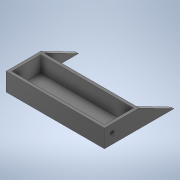
# Autodesk Inventor part: BodyWedgeV1-NoMotor
Saved by Autodesk Inventor 2020 (Build 240168000, 168)
## iProperties
Created: 2023-11-26
Part Number: BodyWedgeV1-NoMotor
Material: Thermoplastic Resin
Document SubType Name: Modeling
Designer: smz3rm
Density: 1.28 g/cm^3
Appearance: Smooth - Black
Mass: 129.558 g
Surface Area: 511.807 cm^2
Volume: 101.217 cm^3
Author: smz3rm
Autodesk Inventor part; units mm, degrees
ref_plane "YZ Plane" through (0, 0, 0) normal (1, 0, 0) x (0, 1, 0)
ref_plane "XZ Plane" through (0, 0, 0) normal (0, 1, 0) x (-1, 0, 0)
ref_plane "XY Plane" through (0, 0, 0) normal (0, 0, 1) x (1, 0, 0)
sketch "Sketch1" plane through (0, 0, 0) normal (0, 1, 0) x (-1, 0, 0)
  line L0 (85, 30) -> (-85, 30)
  line L1 (-85, 30) -> (-85, -30)
  line L2 (-85, -30) -> (85, -30)
  line L3 (85, -30) -> (85, 30)
  line L4 (85, 30) -> (-85, -30) construction
  line L5 (-85, 30) -> (85, -30) construction
  line L6 (0, -42) -> (0, 42) projected
  point P0 (0, 0)
  point P1 (-100, -30)
  point P2 (-85, -27)
  dimension "d0" = 170
  dimension "d1" = 60
  dimension "d32" = 15
  constraints: 12 end point, 2 midpoint, 2 parallel, 2 point on line, 1 horizontal, 1 perpendicular
  measures "d0" distance of L2.end L1.end
  measures "d1" distance of L1.end L0.end
  measures "d32" distance of L1.end point (-100, -30)
extrude "Extrusion1" add sketch "Sketch1" along normal blind 3
sketch "Sketch2" plane through (0, 3, 0) normal (0, 1, 0) x (1, 0, 0)
  line L0 (-85, 30) -> (-85, -30) projected
  line L1 (-85, -30) -> (85, -30) projected
  line L2 (85, -30) -> (85, 30) projected
  line L3 (80, -25) -> (-80, -25)
  line L4 (-80, -25) -> (-80, 25)
  line L5 (-80, 25) -> (80, 25)
  line L6 (80, 25) -> (80, -25)
  line L7 (80, -25) -> (-80, 25) construction
  line L8 (-80, -25) -> (80, 25) construction
  line L9 (85, 30) -> (-85, 30) projected
  point P0 (0, 0)
  dimension "d36" = 160
  dimension "d37" = 50
  constraints: 12 end point, 2 midpoint, 2 parallel, 1 horizontal, 1 perpendicular
  measures "d36" distance of L4.end L5.end
  measures "d37" distance between parallel lines of L5 L3
extrude "Extrusion2" add sketch "Sketch2" along normal blind 28
sketch "Sketch9" plane through (-80, 20, 19) normal (1, 0, 0) x (0, 0, -1)
  circle A0 centre (2, -3) radius 3.5
  line L0 (49, -20) -> (-11, -20) projected
  line L1 (-11, -20) -> (-11, 11) projected
  point P0 (19, -20)
  point P1 (44, -20)
  dimension "d27" = 7
  dimension "d28" = 17
  dimension "d41" = 13
  constraints: 1 centre point
  measures "d27" diameter of A0
  measures "d28" distance from line of L0 A0.centre
  measures "d41" distance from line of L1 A0.centre
extrude "Extrusion7" cut sketch "Sketch9" against normal up to surface (5 mm away)
mirror "Mirror2" about plane through (0, 0, 0) normal (1, 0, 0) of "Extrusion7"
sketch "Sketch14" plane through (0, 3, 0) normal (0, 1, 0) x (1, 0, 0)
  point P0 (0, 0)
sketch "Sketch15" plane through (85, 0, 30) normal (1, 0, 0) x (0, 0, -1)
  line L0 (60, 31) -> (0, 31) projected
  line L1 (60, 31) -> (120, 0)
  line L2 (120, 0) -> (60, 0)
  circle A0 centre (13, 17) radius 3.5 projected
  line L3 (0, 0) -> (60, 0) projected
  line L4 (60, 0) -> (60, 31) projected
  line L5 (0, 31) -> (60, 31) projected
  line L6 (0, 0) -> (0, 31) projected
  point P0 (30, 0)
  dimension "d67" = 60
  constraints: 4 end point, 1 parallel
  measures "d67" distance of L2.end L1.end
extrude "Extrusion12" add sketch "Sketch15" against normal blind 5 contours L1 L2 L4
mirror "Mirror5" about plane through (0, 0, 0) normal (1, 0, 0) of "Extrusion12"
equation "\"d0\" = Width"
equation "\"d1\" = Length"
equation "\"d32\" = -0.5 * Width + 0.5 * FullWidth"
equation "\"d2\" = BaseWallThickness"
equation "\"d36\" = Width - 2 * SideWallThickness"
equation "\"d37\" = Length - 2 * SideWallThickness"
equation "\"d5\" = Height - 2 * BaseWallThickness"
equation "\"d28\" = DriveMotorHeight"
equation "\"d67\" = WedgeLength"
equation "\"d68\" = SideWallThickness"
equation "\"SideWallThickness\" = 5"
equation "\"BaseWallThickness\" = 3"
equation "\"Width\" = 170"
equation "\"Length\" = 60"
equation "\"Height\" = 34"
equation "\"DriveMotorHeight\" = 17"
equation "\"DriveMotorMountThickness\" = 2"
equation "\"WedgeLength\" = 60"
equation "\"FullWidth\" = 200"
body "Solid1"
